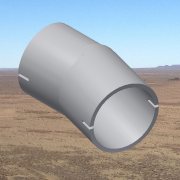
# Autodesk Inventor part: pvc_15bend
Saved by Autodesk Inventor 2013 (Build 170138000, 138)
## iProperties
Created: 2013-07-14
Part Number: pvc_15bend
Material: PVC-Piping
Document SubType Name: Modeling
Designer: ddeboer
Density: 1.4 g/cm^3
Mass: 124.237 g
Surface Area: 466.649 cm^2
Volume: 88.7409 cm^3
Author: ddeboer
Autodesk Inventor part; units mm, degrees
ref_plane "YZ Plane" through (0, 0, 0) normal (1, 0, 0) x (0, 1, 0)
ref_plane "XZ Plane" through (0, 0, 0) normal (0, 1, 0) x (-1, 0, 0)
sketch "Sketch1" plane through (0, 0, 0) normal (1, 0, 0) x (0, 1, 0)
  circle A0 centre (0, 0) radius 30.1625
  circle A1 centre (0, 0) radius 34.0741
  dimension "d0" = 60.325
  dimension "d2" = 3.9116
  constraints: 2 centre point, 1 coincident
  measures "d0" diameter of A0
  measures "d2" radial gap between concentric circles of A1 A0
extrude "Extrusion1" add sketch "Sketch1" along normal blind 50.8
sketch "Sketch2" plane through (50.8, 0, 0) normal (1, 0, 0) x (0, 0, -1)
  circle A0 centre (0, 0) radius 30.1625 projected
  circle A1 centre (0, 0) radius 34.0741 projected
  point P0 (-34.0741, 0)
  constraints: 1 horizontal alignment, 1 other
ref_plane "Work Plane1" through (50.8, 0, 34.0741) normal (0, 0, 1) x (1, 0, 0)
sketch "Sketch3" plane through (50.8, 0, 34.0741) normal (0, 0, 1) x (1, 0, 0)
  line L0 (0.0025, 3.75) -> (0.0025, -3.004)
  point P0 (-50.8, 0)
  constraints: 2 end point, 1 vertical
ref_plane "Work Plane2" through (50.8025, 3.75, 34.0741) normal (-0.9659, 0, -0.2588) x (0, -1, 0)
sketch "Sketch4" plane through (50.8025, 3.75, 34.0741) normal (-0.9659, 0, -0.2588) x (0, -1, 0)
  circle A0 centre (3.75, -33.5383) radius 30.1625
  circle A1 centre (3.75, -33.5383) radius 34.0741
  point P0 (3.75, -19.7644)
  dimension "d6" = 60.325
  dimension "d8" = 3.9116
  constraints: 2 centre point
  measures "d6" diameter of A0
  measures "d8" radial gap between concentric circles of A1 A0
extrude "Extrusion2" add sketch "Sketch4" against normal blind 50.8 and the other way blind 16.51
sketch "Sketch12" plane through (108.5519, 0, 14.8266) normal (0.9659, 0, 0.2588) x (0.2588, 0, -0.9659)
  line L0 (-38.7204, 0) -> (38.3341, 0)
  line L1 (38.3341, 0) -> (38.3341, 2.54)
  line L2 (38.3341, 2.54) -> (-38.7204, 2.54)
  line L3 (-38.7204, 2.54) -> (-38.7204, 0)
  point P0 (-13.7739, 0)
  dimension "d23" = 2.54
  constraints: 8 end point, 2 parallel, 1 horizontal, 1 perpendicular
  measures "d23" distance of L1.end L0.end
extrude "Extrusion5" cut sketch "Sketch12" against normal blind 12.7
sketch "Sketch13" plane through (0, 0, 0) normal (-1, 0, 0) x (0, 0, 1)
  line L0 (-39.4939, 0) -> (40.3288, 0)
  line L1 (40.3288, 0) -> (40.3288, 2.54)
  line L2 (40.3288, 2.54) -> (-39.4939, 2.54)
  line L3 (-39.4939, 2.54) -> (-39.4939, 0)
  dimension "d26" = 2.54
  constraints: 8 end point, 2 parallel, 1 horizontal, 1 perpendicular
  measures "d26" distance of L1.end L0.end
extrude "Extrusion6" cut sketch "Sketch13" against normal blind 12.7
body "Solid1"
